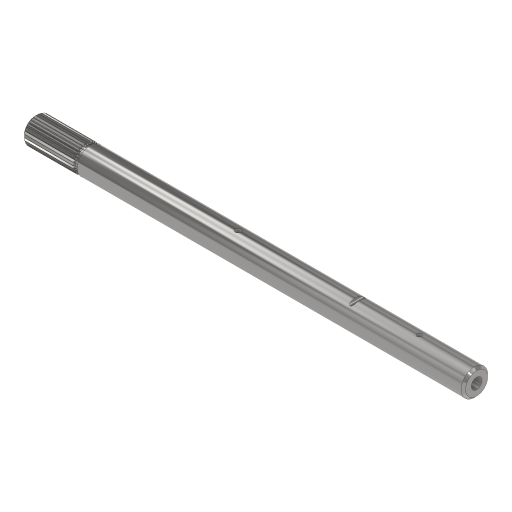
# Autodesk Inventor part: Part026. Grooved shaft
Saved by Autodesk Inventor 2023.2 (Build 272271030, 271C)
## iProperties
Created: 2023-10-07
Part Number: Part026. Grooved shaft
Material: Steel, High Strength, Low Alloy
Document SubType Name: Modeling
Designer: User
Mass: 160.378 g
Surface Area: 99.8222 cm^2
Volume: 20.4303 cm^3
Density: 7.85 g/cm^3
Appearance: Steel - Polished
Author: User
Autodesk Inventor part; units mm, degrees
ref_plane "YZ Plane" through (0, 0, 0) normal (1, 0, 0) x (0, 1, 0)
ref_plane "XZ Plane" through (0, 0, 0) normal (0, 1, 0) x (-1, 0, 0)
sketch "Sketch1" plane through (0, 0, 0) normal (0, 0, 1) x (1, 0, 0)
  line L0 (0, 0) -> (200, 0)
  line L1 (200, 0) -> (200, 6)
  line L2 (200, 6) -> (25, 6)
  line L3 (0, 6) -> (0, 0)
  line L4 (25, 6) -> (25, 5.5)
  line L5 (24.6, 5.1) -> (23.4, 5.1)
  line L6 (23, 5.5) -> (23, 6)
  line L7 (23, 6) -> (0, 6)
  arc A0 (24.6, 5.1) -> (25, 5.5) centre (24.6, 5.5) ccw
  arc A1 (23, 5.5) -> (23.4, 5.1) centre (23.4, 5.5) ccw
  dimension "d0" = 200
  dimension "d1" = 12
  dimension "d2" = 25
  dimension "d3" = 2
  dimension "d4" = 0.9
  dimension "d5" = 0.4
  constraints: 16 end point, 4 parallel, 4 point on circle, 4 tangent, 2 centre point, 1 equal radius, 1 horizontal, 1 perpendicular, 1 point on line
  measures "d0" distance of L3.start L1.end
  measures "d1" diameter of L2 L0
  measures "d2" distance between parallel lines of L4 L3
  measures "d3" distance between parallel lines of L4 L6
  measures "d4" distance between parallel lines of L5 L2
  measures "d5" radius of A0
revolve "Revolution1" add sketch "Sketch1" angle 360 about axis through (0, 0, 0) along (1, 0, 0)
chamfer "Chamfer1" distance 1 angle 45 2 edges at (200, -6, 0) (0, -6, 0)
sketch "Sketch2" plane through (0, 0, 0) normal (-1, 0, 0) x (0, 0, 1)
  circle A0 centre (0, 0) radius 5 construction
  line L0 (-0.5274, 5.9768) -> (-0.0884, 5.1475)
  arc A1 (-0.0884, 5.1475) -> (0.0847, 5.1411) centre (0, 5.1943) ccw
  line L1 (0.0847, 5.1411) -> (0.6044, 5.9695)
  circle A2 centre (0, 0) radius 6 construction
  circle A3 centre (0, 0) radius 5.5 construction
  circle A4 centre (0, 0) radius 5.5 construction
  arc A5 (0.6044, 5.9695) -> (-0.5274, 5.9768) centre (0, 0) ccw
  point P0 (-0.2715, 5.4933)
  point P1 (0.3045, 5.4916)
  dimension "d12" = 11
  dimension "d10" = 60
  dimension "d11" = 0.1
  dimension "d13" = 0.576
  constraints: 6 point on circle, 4 end point, 2 centre point, 2 point on line, 2 tangent, 1 coincident, 1 vertical alignment, 5 other
  measures "d10" angle of L1 L0
  measures "d11" radius of A1
  measures "d13" distance of point (0.305, 5.492) point (-0.271, 5.493)
extrude "Extrusion1" cut sketch "Sketch2" against normal blind 24
pattern_circular "Circular Pattern1" count 30 over 360 about axis through (0.5, 0, 0) along (1, 0, 0) of "Extrusion1"
sketch "Sketch3" plane through (0, 0, 0) normal (0, 0, 1) x (1, 0, 0)
  line L0 (25, 6) -> (199, 6) construction
  circle A0 centre (146, 6) radius 1
  line L1 (200, 5) -> (200, -5) projected
  point P0 (0, 0)
  dimension "d19" = 2
  dimension "d20" = 54
  constraints: 1 centre point, 1 point on line
  measures "d19" diameter of A0
  measures "d20" distance from line of A0.centre L1
extrude "Extrusion2" cut sketch "Sketch3" along normal through all both and the other way through all
sketch "Sketch4" plane through (200, 0, 0) normal (1, 0, 0) x (0, 0, -1)
  circle A0 centre (0, 0) radius 5 projected
  constraints: 1 coincident
hole "Hole1" at (200, 0, 0) direction (-1, 0, 0) diameter 4.8 depth 45 tip angle 118
sketch "Sketch5" plane through (200, 0, 0) normal (1, 0, 0) x (0, 0, -1)
  circle A0 centre (0, 0) radius 5 projected
  constraints: 1 coincident
hole "Hole2" at (200, 0, 0) direction (-1, 0, 0) diameter 4 depth 113 tip angle 118
hole "Hole3" at (92, 6, 0) direction (0, -1, 0) diameter 2.5 depth 6
hole "Hole4" at (174, 6, 0) direction (0, -1, 0) diameter 2 depth 6
ref_plane "Work Plane1" through (92, 0, 0) normal (1, 0, 0) x (0, 0, -1)
ref_plane "Work Plane2" through (174, 0, 0) normal (1, 0, 0) x (0, 0, -1)
body "Solid1"
